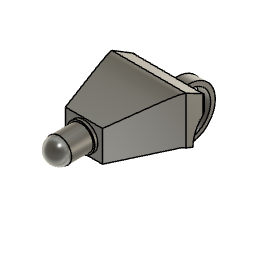
driller v10 (Autodesk Fusion 360 archive; units mm, degrees)
design "arm 1"
Autodesk Fusion 360 part; units mm, degrees
sketch "Sketch3" plane through (0, 0, 0) normal (1, 0, 0) x (0, 1, 0)
  line L0 (-50, 0) -> (-50, 10)
  line L1 (-50, 5) -> (-30, 5) construction
  line L2 (-30, 5) -> (-30, 12.5)
  line L3 (-30, 5) -> (-30, -2.5)
  line L4 (-50, 0) -> (-30, -2.5)
  spline S0 degree 5 poles (-50, 10) (-49.5489, 10.0656) (-48.664, 10.1944) (-47.3883, 10.3797) (-45.7907, 10.6115) (-43.9675, 10.8754) (-42.319, 11.1132) (-40.8452, 11.3249) (-39.544, 11.5107) (-38.4105, 11.671) (-37.4353, 11.8071) (-36.6041, 11.9207) (-35.896, 12.0145) (-35.282, 12.0922) (-34.7245, 12.1586) (-34.1856, 12.2188) (-33.6355, 12.2768) (-33.0591, 12.3345) (-32.4669, 12.3909) (-31.8902, 12.4419) (-31.3646, 12.4829) (-30.9182, 12.5096) (-30.5558, 12.5202) (-30.2523, 12.5161) (-29.9709, 12.5001) (-29.6784, 12.475) (-29.423, 12.4486) (-29.2171, 12.4256) (-29.0734, 12.4088) (-29, 12.4) knots 0 0 0 0 0 0 0.04 0.08 0.12 0.16 0.2 0.24 0.28 0.32 0.36 0.4 0.44 0.48 0.52 0.56 0.6 0.64 0.68 0.72 0.76 0.8 0.84 0.88 0.92 0.96 1 1 1 1 1 1
  circle A0 centre (-18, -4) radius 8.5
  line L5 (-30, -2.5) -> (-26.4995, -4.0904)
  line L6 (-22.1684, 3.4078) -> (-22.1684, 17) construction
  line L7 (-29, 12.4) -> (-23, 9)
  spline S1 degree 5 poles (-23, 9) (-22.97, 8.9744) (-22.9116, 8.925) (-22.8292, 8.8562) (-22.7293, 8.775) (-22.6214, 8.6909) (-22.53, 8.6223) (-22.4541, 8.5661) (-22.3921, 8.5162) (-22.3414, 8.4649) (-22.2997, 8.4053) (-22.2647, 8.3339) (-22.2357, 8.2526) (-22.2123, 8.1658) (-22.1944, 8.0769) (-22.1819, 7.9846) (-22.1739, 7.8811) (-22.1695, 7.7548) (-22.1678, 7.5927) (-22.1677, 7.3832) (-22.1685, 7.1181) (-22.1697, 6.7915) (-22.1708, 6.3996) (-22.1716, 5.9405) (-22.1718, 5.4134) (-22.1714, 4.818) (-22.1705, 4.2875) (-22.1696, 3.8594) (-22.1688, 3.5605) (-22.1684, 3.4078) knots 0 0 0 0 0 0 0.04 0.08 0.12 0.16 0.2 0.24 0.28 0.32 0.36 0.4 0.44 0.48 0.52 0.56 0.6 0.64 0.68 0.72 0.76 0.8 0.84 0.88 0.92 0.96 1 1 1 1 1 1
  circle A1 centre (-18, -4) radius 7
  point P0 (-36, 12)
  point P1 (-33.4, 12.3)
  point P2 (-31.0508, 12.5)
  point P3 (-22.5, 8.6)
  point P4 (-22.3, 8.4)
  point P5 (-22.2, 8.1)
  point P6 (-22.1684, 7.6108)
  dimension "d2" = 10
  dimension "d3" = 20
  dimension "d4" = 7.5
  dimension "d5" = 7.5
  dimension "d6" = 17
  dimension "d7" = 14
  constraint vertical L0
  constraint midpoint L0 L1.start
  constraint perpendicular L0 L1
  constraint perpendicular L1 L2
  constraint perpendicular L1 L3
  constraint coincident A0 L5.end
  constraint coincident A0 L6.start
  constraint vertical L6
  constraint coincident L6 P6
  constraint concentric A0 A1
  measures "d2" distance of L0.start L0.end
  measures "d3" distance of L1.start L1.end
  measures "d4" distance of L1.end L2.end
  measures "d5" distance of L1.end L3.end
  measures "d6" diameter of A0
  measures "d7" diameter of A1
extrude "Extrude1" add sketch "Sketch3" along normal mid plane 24 contours L0 L2 L3 L4 S0 | L2 L3 S0 A0 L5 L7 S1
extrude "Extrude2" add sketch "Sketch3" along normal mid plane 4 contours A0
sketch "Sketch4" plane through (0, 0, 0) normal (1, 0, 0) x (0, 1, 0)
sketch "Sketch5" plane through (0, 0, 0) normal (0, 0, 1) x (1, 0, 0)
  line L0 (0, -50) -> (6, -50) construction
  line L1 (0, -50) -> (-6, -50) construction
  line L2 (-6, -50) -> (-12, -29)
  line L3 (-12, -29) -> (-12, -50)
  line L4 (-12, -50) -> (-6, -50)
  line L5 (12, -29) -> (12, -50)
  line L6 (12, -50) -> (6, -50)
  line L7 (6, -50) -> (12, -29)
  line L8 (12, -29) -> (11.4582, -22.9525)
  line L9 (11.4582, -22.9525) -> (11, -22)
  line L10 (11, -22) -> (12, -22)
  line L11 (12, -22) -> (12, -29)
  line L12 (-12, -29) -> (-12, -22)
  line L13 (-12, -22) -> (-11, -22)
  line L14 (-12, -29) -> (-11.3022, -22.9926)
  line L15 (-11.3022, -22.9926) -> (-11, -22)
  dimension "d12" = 6
  dimension "d13" = 6
  constraint horizontal L0
  constraint parallel L0 L1
  constraint perpendicular L1 L3
  constraint perpendicular L3 L4
  constraint perpendicular L0 L5
  constraint perpendicular L5 L6
  constraint horizontal L10
  constraint perpendicular L10 L11
  constraint parallel L3 L12
  constraint perpendicular L12 L13
  measures "d12" distance of L0.start L0.end
  measures "d13" distance of L0.start L1.end
extrude "Extrude3" cut sketch "Sketch5" along normal blind 13.5 and the other way through all contours L2 L3 L4 | L5 L6 L7
extrude "Extrude4" cut sketch "Sketch5" along normal through all and the other way through all contours L12 L13 L14 L15 | L8 L9 L10 L11
sketch "Sketch6" plane through (0, -50, 0) normal (0, -1, 0) x (1, 0, 0)
  line L0 (-6, 10) -> (-6, 0)
  line L1 (-6, 0) -> (6, 0)
  line L2 (6, 0) -> (6, 10)
  line L3 (6, 10) -> (-6, 10)
  circle A0 centre (0, 5) radius 4.5
  circle A1 centre (0, 5) radius 4
  dimension "d19" = 9
  dimension "d20" = 8
  constraint concentric A0 A1
  measures "d19" diameter of A0
  measures "d20" diameter of A1
extrude "Extrude5" add sketch "Sketch6" along normal blind 12 contours A1
fillet "Fillet1" radius 4 1 edges at (-3.7293, -62, 3.5535)
extrude "Extrude6" add sketch "Sketch6" along normal blind 1 contours A0

design "tire"
Autodesk Fusion 360 part; units mm, degrees
sketch "Sketch1" plane through (0, 0, 0) normal (0, 1, 0) x (1, 0, 0)
  line L0 (0, 0) -> (6, 0) construction
  dimension "d1" = 6
  constraint coincident L0.start origin
  constraint horizontal L0
  measures "d1" distance of L0.start L0.end
sketch "Sketch2" plane through (0, 0, 0) normal (0, 1, 0) x (1, 0, 0)
  line L0 (6, -1) -> (6, -7)
  line L1 (6, -7) -> (8, -7)
  line L2 (8, -7) -> (8, -17)
  line L3 (8, -17) -> (13, -17)
  spline S0 degree 5 poles (13, -17) (13.1944, -16.8351) (13.6033, -16.4449) (14.2764, -15.679) (15.2572, -14.349) (16.4346, -12.3635) (17.1452, -10.6453) (17.4355, -9.3292) (17.5, -8.4443) (17.5, -8) knots 0 0 0 0 0 0 0.2 0.4 0.6 0.8 1 1 1 1 1 1
  line L4 (17.5, -9) -> (17.5, -7)
  line L5 (12.5571, -17.3757) -> (13.4429, -16.6243)
  spline S1 degree 2 poles (17.5, -8) (18.5, -7) (17.3453, -6) knots 0 0 0 0.257413 0.257413 0.257413 weights 1 3 1
  line L6 (17.3453, -6) -> (17.3453, -0.9387)
  line L7 (17.3453, -0.9387) -> (6, -1)
  point P0 (6, 0)
  dimension "d2" = 6
  dimension "d3" = 2
  dimension "d4" = 10
  dimension "d5" = 5
  constraint vertical L0
  constraint perpendicular L0 L1
  constraint perpendicular L1 L2
  constraint coincident L0 P0
  constraint perpendicular L2 L3
  constraint midpoint S0.end L4
  constraint midpoint L3.end L5
  constraint perpendicular L3 L6
  measures "d2" distance of L0.start L0.end
  measures "d3" distance of L0.end L1.end
  measures "d4" distance of L1.end L2.end
  measures "d5" distance of L2.end L3.end
revolve "Revolve1" add sketch "Sketch2" angle 360 about axis through (0, 0, 1.75) along (0, 0, 1)
sketch "Sketch3" plane through (0, 0, 17) normal (0, 0, 1) x (-1, 0, 0)
  circle A0 centre (0, 0) radius 13
  circle A1 centre (0, 0) radius 8
chamfer "Chamfer1" distance 2 angle 45 1 edges at (-7.4586, -2.8929, 17)
sketch "Sketch4" plane through (0, 0, 17) normal (0, 0, 1) x (-1, 0, 0)
sketch "Sketch5" plane through (0, 0, 17) normal (0, 0, 1) x (-1, 0, 0)
sketch "Sketch6" plane through (0, 0, 17) normal (0, 0, 1) x (-1, 0, 0)
  line L0 (-11.8349, -1.75) -> (-11.8349, 1.75)
  line L1 (0, 0) -> (-11.8349, 0) construction
  line L2 (-11.8349, -1.75) -> (-16.1651, -4.25)
  line L3 (-11.8349, 1.75) -> (-16.1651, 4.25)
  arc A0 (-16.1651, 4.25) -> (-16.1651, -4.25) centre (-5.7658, 0) ccw
  dimension "d18" = 5
  dimension "d19" = 120
  dimension "d20" = 5
  dimension "d21" = 120
  constraint vertical L0
  constraint coincident L1.start origin
  constraint midpoint L0 L1.end
  constraint perpendicular L0 L1
  measures "d18" distance of L0.start L2.end
  measures "d19" angle of L0 L2
  measures "d20" distance of L0.end L3.end
  measures "d21" angle of L0 L3
extrude "Extrude1" cut sketch "Sketch6" against normal blind 6
sketch "Sketch7" plane through (0, 0, 17) normal (0, 0, 1) x (-1, 0, 0)
pattern_circular "C-Pattern2" count 7 over 360 about axis through (0, 0, 1.75) along (0, 0, 1) of "Extrude1"

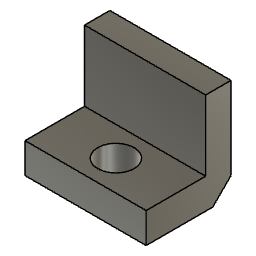
design "seat"
Autodesk Fusion 360 part; units mm, degrees
sketch "Sketch1" plane through (0, 0, 0) normal (1, 0, 0) x (0, 1, 0)
  line L0 (-25, 25) -> (-11, 25)
  line L1 (-11, 25) -> (-11, 23)
  line L2 (-14, 20) -> (-25, 20)
  line L3 (-25, 20) -> (-25, 25)
  line L4 (-14, 20) -> (-15.1746, 20)
  line L5 (-15.1746, 20) -> (-15.1746, 36.6158)
  line L6 (-15.1746, 36.6158) -> (-11, 36.6158)
  line L7 (-11, 36.6158) -> (-11, 23)
  line L8 (-14, 20) -> (-11, 23)
  dimension "d1" = 14
  constraint horizontal L0
  constraint vertical L1
  constraint horizontal L2
  constraint vertical L3
  constraint horizontal L4
  constraint vertical L5
  constraint horizontal L6
  constraint vertical L7
  measures "d1" distance of L0.start L0.end
extrude "Extrude1" add sketch "Sketch1" along normal blind 20
sketch "Sketch2" plane through (0, 0, 25) normal (0, 0, 1) x (-1, 0, 0)
  line L0 (0, 15.1746) -> (0, 25)
  line L1 (0, 25) -> (-20, 25)
  line L2 (-20, 25) -> (-20, 15.1746)
  line L3 (-20, 15.1746) -> (0, 15.1746)
  circle A0 centre (-10, 20) radius 3
  dimension "d5" = 6
  measures "d5" diameter of A0
extrude "Extrude2" cut sketch "Sketch2" against normal blind 65 contours A0

design "screw"
Autodesk Fusion 360 part; units mm, degrees
sketch "Sketch1" plane through (0, 0, 0) normal (0, 0, 1) x (1, 0, 0)
  circle A0 centre (0, 0) radius 7
  circle A1 centre (0, 0) radius 6
  circle A2 centre (0, 0) radius 3.5
  dimension "d3" = 14
  dimension "d4" = 12
  dimension "d5" = 7
  constraint coincident A0.centre A1.centre
  constraint concentric A0 A1
  constraint concentric A1 A2
  measures "d3" diameter of A0
  measures "d4" diameter of A1
  measures "d5" diameter of A2
extrude "Extrude1" add sketch "Sketch1" along normal blind 1 contours A0
sketch "Sketch2" plane through (0, 0, 0) normal (0, 0, 1) x (1, 0, 0)
  circle A0 centre (0, 0) radius 6
  circle A1 centre (0, 0) radius 3.5
  dimension "d8" = 12
  dimension "d9" = 7
  constraint coincident A0.centre A1.centre
  measures "d8" diameter of A0
  measures "d9" diameter of A1
extrude "Extrude2" add sketch "Sketch2" along normal blind 5 contours A0 | A1
sketch "Sketch3" plane through (0, 0, 5) normal (0, 0, 1) x (-1, 0, 0)
  circle A0 centre (0, 0) radius 6
  line L0 (-4, -1) -> (4, -1)
  line L1 (4, -1) -> (4, 1)
  line L2 (4, 1) -> (-4, 1)
  line L3 (-4, 1) -> (-4, -1)
  line L4 (-4, -1) -> (4, 1) construction
  line L5 (4, -1) -> (-4, 1) construction
  dimension "d12" = 8
  constraint horizontal L0
  constraint perpendicular L0 L1
  constraint parallel L0 L2
  constraint parallel L1 L3
  constraint coincident L4 A0.centre
  constraint coincident L5 A0.centre
  constraint coincident A0.centre origin
  measures "d12" distance of L1.end L2.end
extrude "Extrude3" cut sketch "Sketch3" against normal blind 3 contours L0 L1 L2 L3
pattern_circular "C-Pattern1" count 4 over 360 about axis through (0, 0, 1.75) along (0, 0, 1) of "Extrude3"
sketch "Sketch4" plane through (0, 0, 0) normal (0, 0, 1) x (1, 0, 0)
  circle A0 centre (0, 0) radius 4.5
  dimension "d17" = 9
  constraint coincident A0.centre origin
  measures "d17" diameter of A0
fillet "Fillet1" radius 4 1 edges at (-5.594, -2.1697, 5)
sketch "Sketch5" plane through (0, 0, 0) normal (0, 0, -1) x (1, 0, 0)
  circle A0 centre (0, 0) radius 7
  circle A1 centre (0, 0) radius 4.5
  dimension "d22" = 9
  measures "d22" diameter of A1
sketch "Sketch6" plane through (0, 0, 0) normal (1, 0, 0) x (0, 1, 0)
sketch "Sketch7" plane through (0, 0, 0) normal (0, 0, -1) x (1, 0, 0)
  circle A0 centre (0, 0) radius 7
  circle A1 centre (0, 0) radius 3
  dimension "d25" = 6
  measures "d25" diameter of A1
extrude "Extrude6" add sketch "Sketch7" along normal blind 14 contours A1
delete_face "DeleteFace1" 1 faces at (2.9851, 0.2987, -9.3333)
extrude "Extrude7" add sketch "Sketch7" along normal blind 13 contours A1
thread "Thread2" [suppressed]

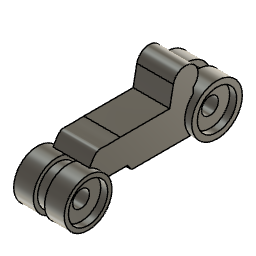
design "arm 2"
Autodesk Fusion 360 part; units mm, degrees
sketch "Sketch1" plane through (0, 0, 0) normal (1, 0, 0) x (0, 1, 0)
  circle A0 centre (0, 0) radius 8.5
  circle A1 centre (0, 0) radius 7
  line L0 (1.2528, 12) -> (30.2528, 12) construction
  spline S0 degree 5 poles (3.0055, 7.9509) (3.0882, 8.099) (3.2479, 8.3834) (3.4706, 8.7746) (3.7337, 9.2254) (4.0071, 9.6726) (4.2299, 10.0129) (4.4123, 10.2664) (4.5733, 10.4708) (4.7414, 10.6811) (4.9475, 10.9417) (5.22, 11.2652) (5.5777, 11.6027) (6.0307, 11.8739) (6.5823, 12.0162) (7.2303, 12.0075) (7.9673, 11.9482) (8.787, 11.9001) (9.6843, 11.887) (10.655, 11.9095) (11.6962, 11.9519) (12.584, 11.9836) (13.2803, 11.997) (13.7578, 12) (14, 12) knots 0 0 0 0 0 0 0.05 0.1 0.15 0.2 0.25 0.3 0.35 0.4 0.45 0.5 0.55 0.6 0.65 0.7 0.75 0.8 0.85 0.9 0.95 1 1 1 1 1 1
  line L1 (12.2472, 12) -> (15.7528, 12)
  line L2 (5.8541, 12) -> (8.1459, 12)
  line L3 (14, 12) -> (14, 2) construction
  line L4 (8.5, 0.0081) -> (9.1, 1.5)
  spline S1 degree 5 poles (9.1, 1.5) (9.1101, 1.5172) (9.1298, 1.5505) (9.1581, 1.5975) (9.1933, 1.6541) (9.233, 1.7146) (9.2691, 1.7647) (9.3025, 1.8048) (9.3352, 1.8357) (9.3704, 1.8592) (9.4118, 1.8773) (9.4632, 1.8924) (9.5279, 1.9065) (9.6083, 1.9212) (9.7052, 1.9375) (9.819, 1.9559) (9.9232, 1.9724) (10.0088, 1.9858) (10.0691, 1.9952) (10.1, 2) knots 0 0 0 0 0 0 0.066667 0.133333 0.2 0.266667 0.333333 0.4 0.466667 0.533333 0.6 0.666667 0.733333 0.8 0.866667 0.933333 1 1 1 1 1 1
  line L5 (0, 0) -> (46, 0) construction
  circle A2 centre (45.9282, 5.7446) radius 9
  circle A3 centre (45.9282, 5.7446) radius 7
  line L6 (10.1, 2) -> (16.5, 2)
  line L7 (16.5, 2) -> (18, 0)
  line L8 (18, 0) -> (39, 0)
  line L9 (14, 12) -> (31.5582, 12)
  line L10 (39.9718, 12.4915) -> (39.9718, 14.5)
  circle A4 centre (37.2359, 18) radius 4.4424
  line L11 (31.5582, 12) -> (32.8734, 18.839)
  point P0 (4.3699, 10.204)
  point P1 (5, 11)
  point P2 (7, 12)
  point P3 (9.3, 1.8)
  point P4 (9.5, 1.9)
  dimension "d1" = 17
  dimension "d2" = 14
  dimension "d3" = 10
  dimension "d4" = 46
  dimension "d5" = 18
  dimension "d6" = 14
  constraint coincident A0.centre A1.centre
  constraint horizontal L0
  constraint coincident L0 P2
  constraint coincident L0 S0.end
  constraint midpoint S0.end L1
  constraint midpoint L0 L1.end
  constraint midpoint P2 L2
  constraint coincident L0 L2.end
  constraint perpendicular L0 L3
  constraint coincident A0 S0.start
  constraint coincident A0 L4.start
  constraint horizontal L5
  constraint concentric A2 A3
  constraint perpendicular L3 L6
  constraint coincident L5 L7.end
  constraint coincident L5 L8.end
  constraint coincident A2 L8.end
  constraint coincident A2 L10.start
  constraint vertical L10
  constraint coincident L10.end A4
  constraint coincident A4 L11.end
  constraint tangent A4 L11
  measures "d1" diameter of A0
  measures "d2" diameter of A1
  measures "d3" distance of S0.end L3.end
  measures "d4" distance of A0.centre L5.end
  measures "d5" diameter of A2
  measures "d6" diameter of A3
sketch "Sketch2" plane through (0, 0, 0) normal (1, 0, 0) x (0, 1, 0)
  line L0 (8.5, 0) -> (9.5, 1.5)
  spline S0 degree 5 poles (9.5, 1.5) (9.5153, 1.5208) (9.5459, 1.5616) (9.592, 1.6199) (9.6538, 1.6919) (9.7318, 1.7718) (9.8106, 1.8405) (9.8901, 1.8972) (9.9705, 1.9412) (10.0518, 1.9728) (10.1338, 1.993) (10.1999, 2.0007) (10.2498, 2.0021) (10.2833, 2.001) (10.3, 2) knots 0 0 0 0 0 0 0.1 0.2 0.3 0.4 0.5 0.6 0.7 0.8 0.9 1 1 1 1 1 1
  line L1 (10.3, 2) -> (14, 2)
  circle A0 centre (0, 0) radius 3
  circle A1 centre (45.9282, 5.7446) radius 3
  circle A2 centre (45.9282, 5.7446) radius 7
  circle A3 centre (0, 0) radius 7
  point P0 (9.9, 1.9)
  point P1 (45.9282, 5.7446)
  dimension "d13" = 6
  dimension "d14" = 6
  dimension "d15" = 14
  dimension "d16" = 14
  constraint horizontal L1
  constraint coincident A0.centre A3.centre
  constraint coincident P1 A1.centre
  constraint concentric A1 A2
  measures "d13" diameter of A0
  measures "d14" diameter of A1
  measures "d15" diameter of A2
  measures "d16" diameter of A3
extrude "Extrude1" add sketch "Sketch1" along normal mid plane 13 contours A0 S0 L1 L4 S1 A2 L6 L7 L8 L9 L10 A4 L11 | A4
extrude "Extrude2" add sketch "Sketch1" along normal mid plane 18 contours A0 | A2
sketch "Sketch3" plane through (0, 0, 0) normal (1, 0, 0) x (0, 1, 0)
sketch "Sketch4" plane through (0, 0, 0) normal (1, 0, 0) x (0, 1, 0)
sketch "Sketch5" plane through (0, 0, 0) normal (1, 0, 0) x (0, 1, 0)
extrude "Extrude3" cut sketch "Sketch1" along normal mid plane 4 contours A0 | A2
extrude "Extrude4" add sketch "Sketch1" along normal mid plane 13 contours A1
extrude "Extrude5" add sketch "Sketch2" along normal mid plane 13 contours A2
extrude "Extrude6" cut sketch "Sketch2" along normal mid plane 13 contours A0

design "arm base"
Autodesk Fusion 360 part; units mm, degrees
sketch "Sketch1" plane through (0, 0, 0) normal (1, 0, 0) x (0, 1, 0)
  line L0 (-20, 20) -> (-7, 20)
  line L1 (-20, 20) -> (-27.566, 12.434)
  line L2 (-27.566, 12.434) -> (-27.566, 2.434)
  line L3 (-27.566, 2.434) -> (-30, 2.434)
  line L4 (-30, 2.434) -> (-30, 14)
  line L5 (-30, 14) -> (-24, 20)
  line L6 (-24, 20) -> (-21, 20)
  line L7 (-21, 20) -> (-21, 19)
  line L8 (-29.5, 14.5) -> (-29.5, 20)
  line L9 (-26.5, 23) -> (-7, 23)
  line L10 (-7, 20) -> (-7, 23)
  arc A0 (-26.5, 23) -> (-29.5, 20) centre (-26.5, 20) ccw
  dimension "d1" = 13
  dimension "d2" = 10.7
  dimension "d3" = 10
  dimension "d4" = 3
  constraint horizontal L0
  constraint vertical L2
  constraint perpendicular L2 L3
  constraint perpendicular L3 L4
  constraint perpendicular L2 L6
  constraint coincident L1 L7.end
  constraint vertical L7
  constraint coincident L5 L8.start
  constraint perpendicular L0 L8
  constraint perpendicular L8 L9
  constraint tangent L8 A0
  constraint tangent L9 A0
  measures "d1" distance of L0.start L0.end
  measures "d2" distance of L0.start L1.end
  measures "d3" distance of L1.end L2.end
  measures "d4" radius of A0
extrude "Extrude1" add sketch "Sketch1" along normal mid plane 24 makes body 1
extrude "Extrude2" add sketch "Sketch1" along normal mid plane 27 separate body contours L1 L2 L3 L4 L5 L6 L7 makes body 2
sketch "Sketch2" plane through (0, 0, 23) normal (0, 0, 1) x (-1, 0, 0)
  line L0 (12, 26.5) -> (-12, 26.5)
  line L1 (-12, 26.5) -> (-12, 7)
  line L2 (-12, 7) -> (12, 7)
  line L3 (12, 7) -> (12, 26.5)
  line L4 (12, 14.5) -> (12, 7)
  line L5 (-12, 7) -> (-12, 14.5)
  arc A0 (12, 14.5) -> (-12, 14.5) centre (0, 14.5) ccw
  constraint coincident L2.end L3.start
  constraint coincident L1.end L2.start
  constraint tangent L5 A0
extrude "Extrude3" add sketch "Sketch2" along normal blind 3 contours L1 L2 L3 L4 L5 A0 bodies 1
fillet "Fillet1" radius 3 3 edges at (-12, -10.75, 26) (0, -26.5, 26) (12, -10.75, 26) on bodies 1
extrude "Extrude4" cut 1 faces at (-0.6676, -17.4248, 26) along direction (0, 0, -1) blind 3 on bodies 1 bodies 1
sketch "Sketch3" plane through (0, 0, 23) normal (0, 0, 1) x (-1, 0, 0)
  line L0 (-9, 14.5) -> (-9, 7)
  line L1 (-9, 7) -> (9, 7)
  line L2 (9, 7) -> (9, 14.5)
  arc A0 (9, 14.5) -> (-9, 14.5) centre (0, 14.5) ccw
  circle A1 centre (0, 15) radius 5.5
  dimension "d15" = 11
  measures "d15" diameter of A1
extrude "Extrude5" cut sketch "Sketch3" against normal through all contours A1 bodies 1
sketch "Sketch4" plane through (12, 0, 0) normal (1, 0, 0) x (0, 1, 0)
  line L0 (-20, 20) -> (-7, 20)
  line L1 (-7, 20) -> (-7, 23)
  line L2 (-7, 23) -> (-14.5, 23)
  line L3 (-14.5, 23) -> (-26.5, 23)
  arc A0 (-26.5, 23) -> (-29.5, 20) centre (-26.5, 20) ccw
  line L4 (-29.5, 20) -> (-29.5, 14.5)
  line L5 (-29.5, 14.5) -> (-30, 14)
  line L6 (-30, 14) -> (-30, 2.434)
  line L7 (-30, 2.434) -> (-27.566, 2.434)
  line L8 (-27.566, 2.434) -> (-27.566, 12.434)
  line L9 (-27.566, 12.434) -> (-20, 20)
  line L10 (-20, 20) -> (-20, 34) construction
  constraint coincident L0.start L9.end
  constraint perpendicular L0 L10
sketch "Sketch5" plane through (0, 0, 0) normal (0, 0, 1) x (1, 0, 0)
  line L0 (0, -15, 23) -> (12, -15, 23) construction
  line L1 (0, -15, 23) -> (-12, -15, 23) construction
sketch "Sketch6" plane through (12, 0, 0) normal (1, 0, 0) x (0, 1, 0)
sketch "Sketch7" plane through (0, 0, 23) normal (0, 0, 1) x (-1, 0, 0)
sketch "Sketch8" plane through (12, 0, 0) normal (1, 0, 0) x (0, 1, 0)
  line L0 (-15, 23) -> (-15, 20) construction
  line L1 (-15, 20) -> (-20, 20) construction
  constraint vertical L0
  constraint perpendicular L0 L1
sketch "Sketch9" plane through (12, 0, 0) normal (1, 0, 0) x (0, 1, 0)
  line L0 (-13, 20) -> (-13, 23)
  arc A0 (-13, 23) -> (-15, 23) centre (-14, 23) ccw
  line L1 (-15, 23) -> (-15, 20)
  line L2 (-15, 20) -> (-13, 20)
  constraint tangent L0 A0
  constraint tangent A0 L1
  constraint vertical L1
sketch "Sketch11" plane through (-12, 0, 0) normal (-1, 0, 0) x (0, -1, 0)
  line L0 (7, 20) -> (20, 20)
  line L1 (20, 20) -> (27.566, 12.434)
  line L2 (27.566, 12.434) -> (27.566, 2.434)
  line L3 (27.566, 2.434) -> (30, 2.434)
  line L4 (30, 2.434) -> (30, 14)
  line L5 (30, 14) -> (29.5, 14.5)
  line L6 (29.5, 14.5) -> (29.5, 20)
  arc A0 (29.5, 20) -> (26.5, 23) centre (26.5, 20) ccw
  line L7 (26.5, 23) -> (14.5, 23)
  line L8 (14.5, 23) -> (7, 23)
  line L9 (7, 23) -> (7, 20)
  line L10 (15, 23) -> (15, 20)
  line L11 (12.9998, 23) -> (12.9998, 20)
  line L12 (15, 20) -> (12.9998, 20)
  arc A1 (15, 23) -> (12.9998, 23) centre (13.9999, 23) ccw
  line L13 (15, 22) -> (12.9998, 22) construction
  constraint coincident L7 L10.start
  constraint coincident L0 L10.end
  constraint perpendicular L0 L10
  constraint coincident L8 L11.start
  constraint coincident L0 L11.end
  constraint perpendicular L0 L11
  constraint perpendicular L11 L12
  constraint tangent L10 A1
  constraint coincident L10 L13.start
  constraint coincident L11 L13.end
  constraint perpendicular L11 L13
extrude "Extrude6" cut sketch "Sketch9" against normal blind 2 bodies 1
extrude "Extrude7" cut sketch "Sketch11" against normal blind 2 contours L0 L7 L8 L10 L11 L12 | L7 L8 A1 bodies 1

design "main body"
Autodesk Fusion 360 part; units mm, degrees
sketch "Sketch1" plane through (0, 0, 0) normal (1, 0, 0) x (0, 1, 0)
  line L0 (36, 12.5) -> (-36, 12.5)
  line L1 (-43.5, 5) -> (-43.5, -7.5)
  line L2 (-38.5, -12.5) -> (38.5, -12.5)
  line L3 (43.5, -7.5) -> (43.5, 5)
  line L4 (43.5, 12.5) -> (-43.5, -12.5) construction
  line L5 (-43.5, 12.5) -> (43.5, -12.5) construction
  line L6 (-36, 12.5) -> (-43.5, 5)
  line L7 (36, 12.5) -> (43.5, 5)
  line L8 (-38.5, -12.5) -> (-43.5, -7.5)
  line L9 (43.5, -7.5) -> (38.5, -12.5)
  line L10 (-43.5, -5.0494) -> (43.5, -5.0494) construction
  dimension "d1" = 87
  dimension "d2" = 25
  dimension "d3" = 7.5
  dimension "d4" = 7.5
  dimension "d5" = 7.5
  dimension "d6" = 7.5
  dimension "d7" = 5
  dimension "d8" = 5
  dimension "d9" = 5
  dimension "d10" = 5
  constraint horizontal L0
  constraint perpendicular L0 L1
  constraint parallel L0 L2
  constraint parallel L1 L3
  constraint coincident L4 origin
  constraint coincident L5 origin
  constraint coincident L5.start L0
  constraint coincident L5.start L1
  constraint coincident L4.start L0
  constraint coincident L4.start L3
  constraint coincident L4.end L2
  constraint coincident L4.end L1
  constraint coincident L5.end L3
  constraint coincident L5.end L2
  constraint coincident L1 L10.start
  constraint coincident L3 L10.end
  constraint perpendicular L3 L10
  measures "d1" distance of L4.end L5.end
  measures "d2" distance of L5.start L4.end
  measures "d3" distance of L5.start L0.end
  measures "d4" distance of L5.start L1.start
  measures "d5" distance of L4.start L0.start
  measures "d6" distance of L4.start L3.end
  measures "d7" distance of L4.end L2.start
  measures "d8" distance of L4.end L1.end
  measures "d9" distance of L5.end L3.start
  measures "d10" distance of L5.end L2.end
extrude "Extrude1" add sketch "Sketch1" along normal mid plane 27
sketch "Sketch2" plane through (-13.5, 0, 0) normal (-1, 0, 0) x (0, -1, 0)
  line L0 (36, 12.5) -> (-36, 12.5)
  line L1 (-36, 12.5) -> (-43.5, 5)
  line L2 (-43.5, 5) -> (-43.5, -7.5)
  line L3 (-43.5, -7.5) -> (-38.5, -12.5)
  line L4 (-38.5, -12.5) -> (38.5, -12.5)
  line L5 (38.5, -12.5) -> (43.5, -7.5)
  line L6 (43.5, -7.5) -> (43.5, 5)
  line L7 (43.5, 5) -> (36, 12.5)
  circle A0 centre (-30, -5) radius 5.5
  circle A1 centre (30, -5) radius 5.5
  circle A2 centre (30, -5) radius 3
  circle A3 centre (-30, -5) radius 3
  dimension "d13" = 11
  dimension "d14" = 11
  dimension "d15" = 6
  dimension "d16" = 6
  constraint concentric A1 A2
  constraint concentric A0 A3
  measures "d13" diameter of A0
  measures "d14" diameter of A1
  measures "d15" diameter of A2
  measures "d16" diameter of A3
sketch "Sketch4" plane through (13.5, 0, 0) normal (1, 0, 0) x (0, 1, 0)
  line L0 (36, 12.5) -> (-36, 12.5)
  line L1 (-36, 12.5) -> (-43.5, 5)
  line L2 (-43.5, 5) -> (-43.5, -7.5)
  line L3 (-43.5, -7.5) -> (-38.5, -12.5)
  line L4 (-38.5, -12.5) -> (38.5, -12.5)
  line L5 (38.5, -12.5) -> (43.5, -7.5)
  line L6 (43.5, -7.5) -> (43.5, 5)
  line L7 (43.5, 5) -> (36, 12.5)
  circle A0 centre (-30, -5) radius 5.5
  circle A1 centre (-30, -5) radius 3
  circle A2 centre (30, -5) radius 5.5
  circle A3 centre (30, -5) radius 3
  dimension "d17" = 11
  dimension "d18" = 6
  dimension "d19" = 11
  dimension "d20" = 6
  constraint concentric A0 A1
  constraint concentric A2 A3
  measures "d17" diameter of A0
  measures "d18" diameter of A1
  measures "d19" diameter of A2
  measures "d20" diameter of A3
extrude "Extrude2" add sketch "Sketch2" along normal blind 7 contours A0 | A1
extrude "Extrude3" add sketch "Sketch4" along normal blind 7 contours A0 | A2
sketch "Sketch5" plane through (0, 0, 0) normal (1, 0, 0) x (0, 1, 0)
  line L0 (36, 13) -> (23, 13) construction
  line L1 (43.5, 5) -> (-43.5, 5) construction
  line L2 (20, 13) -> (-20, 13) construction
  line L3 (-23, 5) -> (-36, 5) construction
  constraint horizontal L0
  constraint horizontal L1
  constraint horizontal L2
  constraint horizontal L3
sketch "Sketch6" plane through (0, 0, 0) normal (1, 0, 0) x (0, 1, 0)
  line L0 (28, 5) -> (28, -5) construction
  constraint vertical L0
sketch "Sketch7" plane through (0, 0, 12.5) normal (0, 0, 1) x (-1, 0, 0)
  line L0 (13.5, 36) -> (-13.5, 36)
  line L1 (-13.5, 36) -> (-13.5, -36)
  line L2 (-13.5, -36) -> (13.5, -36)
  line L3 (13.5, -36) -> (13.5, 36)
  line L4 (12, 30) -> (-12, 30) construction
  line L5 (13.5, 35.0128) -> (-13.5, 35.0128) construction
  constraint perpendicular L3 L4
  constraint coincident L3 L5.start
  constraint coincident L1 L5.end
  constraint perpendicular L1 L5
sketch "Sketch8" plane through (0, 0, 12.5) normal (0, 0, 1) x (1, 0, 0)
sketch "Sketch9" plane through (0, 0, 0) normal (1, 0, 0) x (0, 1, 0)
sketch "Sketch10" plane through (0, 0, 12.5) normal (0, 0, 1) x (-1, 0, 0)
sketch "Sketch11" plane through (0, 0, 0) normal (1, 0, 0) x (0, 1, 0)
  line L0 (-36, 12.5) -> (-31, 12.5) construction
  dimension "d26" = 5
  constraint horizontal L0
  measures "d26" distance of L0.start L0.end
sketch "Sketch12" plane through (0, 0, 12.5) normal (0, 0, 1) x (-1, 0, 0)
  circle A0 centre (0, 31) radius 3
  dimension "d27" = 6
  measures "d27" diameter of A0
sketch "Sketch13" plane through (0, 0, 12.5) normal (0, 0, 1) x (1, 0, 0)
sketch "Sketch14" plane through (0, 0, 0) normal (1, 0, 0) x (0, 1, 0)
  line L0 (-0.5, 12.5) -> (-0.5, -12.5) construction
  line L1 (-0.5, 12.5) -> (-0.5, 47.5) construction
  dimension "d28" = 35
  constraint vertical L0
  constraint parallel L0 L1
  measures "d28" distance of L0.start L1.end
sketch "Sketch16" plane through (0, 0, 12.5) normal (0, 0, 1) x (-1, 0, 0)
  circle A0 centre (0, 0) radius 3
  circle A1 centre (0, -30) radius 3
  dimension "d29" = 6
  dimension "d30" = 6
  constraint coincident A0.centre origin
  measures "d29" diameter of A0
  measures "d30" diameter of A1
extrude "Extrude4" cut sketch "Sketch12" against normal blind 20
extrude "Extrude5" cut sketch "Sketch16" against normal blind 5
sketch "Sketch17" plane through (0, 0, -12.5) normal (0, 0, -1) x (1, 0, 0)
  line L0 (-13.5, -38.5) -> (13.5, -38.5)
  line L1 (13.5, -38.5) -> (13.5, 38.5)
  line L2 (13.5, 38.5) -> (-13.5, 38.5)
  line L3 (-13.5, 38.5) -> (-13.5, -38.5)
  line L4 (7.5745, -30) -> (7.5745, 5.0261)
  line L5 (-8, -30) -> (-8, 5)
  arc A0 (-8, -30) -> (7.5745, -30) centre (-0.2127, -30) ccw
  arc A1 (7.5745, 5.0261) -> (-8, 5) centre (-0.2128, 5.0261) ccw
  constraint parallel L1 L4
  constraint perpendicular L0 L5
  constraint tangent L5 A0
  constraint tangent L4 A0
  constraint tangent L4 A1
extrude "Extrude6" cut sketch "Sketch17" against normal blind 20 contours L4 L5 A0 A1
sketch "Sketch18" plane through (0, 0, 12.5) normal (0, 0, 1) x (-1, 0, 0)
  circle A0 centre (0, -30) radius 3
  circle A1 centre (0, 0) radius 3
  circle A2 centre (0, 31) radius 3
  line L0 (13.5, 36) -> (-13.5, 36)
  line L1 (-13.5, 36) -> (-13.5, -36)
  line L2 (-13.5, -36) -> (13.5, -36)
  line L3 (13.5, -36) -> (13.5, 36)
  line L4 (5, 43.5) -> (-5, 43.5)
  line L5 (-5, 43.5) -> (-5, 38.5)
  line L6 (-5, 38.5) -> (5, 38.5)
  line L7 (5, 38.5) -> (5, 43.5)
  constraint horizontal L4
  constraint vertical L5
  constraint horizontal L6
  constraint vertical L7
extrude "Extrude7" cut sketch "Sketch18" against normal blind 10 contours L4 L5 L6 L7
sketch "Sketch19" plane through (0, 0, 12.5) normal (0, 0, 1) x (-1, 0, 0)
  circle A0 centre (0, -30) radius 3
  dimension "d41" = 6
  measures "d41" diameter of A0
sketch "Sketch20" plane through (0, 0, 12.5) normal (0, 0, 1) x (-1, 0, 0)
  circle A0 centre (0, 31) radius 3.5
  dimension "d47" = 7
  measures "d47" diameter of A0
equation "d4 = d3"
equation "d6 = d5"
equation "d8 = d7"
equation "d10 = d9"
